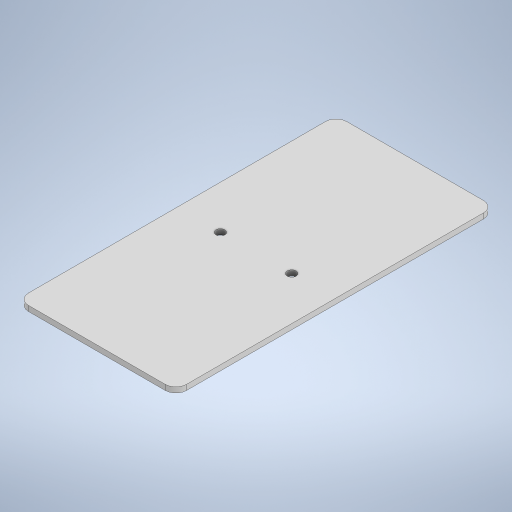
# Autodesk Inventor part: Pedana
Saved by Autodesk Inventor 2024 (Build 280153000, 153)
## iProperties
Created: 2023-11-20
Part Number: Pedana
Material: Generico
Document SubType Name: Modeling
Designer: Leonardo
Density: 1 g/cm^3
Appearance: Default
Author: Leonardo
Autodesk Inventor part; units mm, degrees
ref_plane "YZ Plane" through (0, 0, 0) normal (1, 0, 0) x (0, 1, 0)
ref_plane "XZ Plane" through (0, 0, 0) normal (0, 1, 0) x (-1, 0, 0)
ref_plane "XY Plane" through (0, 0, 0) normal (0, 0, 1) x (1, 0, 0)
sketch "Schizzo_pedana" plane through (0, 0, 0) normal (0, 1, 0) x (-1, 0, 0)
  line L0 (-20, 0) -> (-20, 280)
  line L1 (278, 0) -> (278, 280)
  line L2 (258, 300) -> (0, 300)
  line L3 (278, 0) -> (278, -280)
  line L4 (-20, 0) -> (-20, -280)
  line L5 (0, -300) -> (258, -300)
  circle A0 centre (196.1614, 0) radius 8.5276
  circle A1 centre (61.6876, 0) radius 8.634
  arc A2 (258, -300) -> (278, -280) centre (258, -280) ccw
  arc A3 (-20, -280) -> (0, -300) centre (0, -280) ccw
  arc A4 (0, 300) -> (-20, 280) centre (0, 280) ccw
  arc A5 (278, 280) -> (258, 300) centre (258, 280) ccw
  point P0 (0, 0)
  point P1 (-20, 300)
  point P2 (278, 300)
  point P3 (278, -300)
  point P4 (-20, -300)
  dimension "d7" = 300
  dimension "d10" = 300
  dimension "d13" = 20
  dimension "d14" = 20
  constraints: 12 end point, 8 point on circle, 8 point on line, 8 tangent, 6 centre point, 4 vertical, 2 equal radius, 1 perpendicular
  measures "d7" distance of L0.start point (-20, 300)
  measures "d10" distance of L0.start point (-20, -300)
  measures "d13" radius of A2
  measures "d14" radius of A3
extrude "Estrusione2" add sketch "Schizzo_pedana" along normal blind 10
